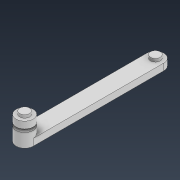
# Autodesk Inventor part: Support
Saved by Autodesk Inventor 2021 (Build 250183000, 183)
## iProperties
Created: 2021-01-30
Part Number: Support
Material: Generic
Document SubType Name: Modeling
Designer: PaisW
Density: 1 g/cm^3
Appearance: Default
Author: PaisW
Autodesk Inventor part; units mm, degrees
ref_plane "YZ Plane" through (0, 0, 0) normal (1, 0, 0) x (0, 1, 0)
ref_plane "XZ Plane" through (0, 0, 0) normal (0, 1, 0) x (-1, 0, 0)
ref_plane "XY Plane" through (0, 0, 0) normal (0, 0, 1) x (1, 0, 0)
sketch "Sketch1" plane through (0, 0, 0) normal (0, 1, 0) x (-1, 0, 0)
  line L0 (26.15, 200) -> (-26.15, 200)
  line L1 (-26.15, 200) -> (-26.15, -200)
  line L2 (-26.15, -200) -> (26.15, -200)
  line L3 (26.15, -200) -> (26.15, 200)
  circle A0 centre (0, 200) radius 26.15
  circle A1 centre (0, -200) radius 26.15
  point P0 (0, 0)
  point P1 (26.15, 0)
  point P2 (26.15, 200)
  point P3 (26.15, -200)
  dimension "d0" = 52.3
  dimension "d1" = 400
  constraints: 8 end point, 3 midpoint, 2 parallel, 1 coincident, 1 horizontal, 1 horizontal alignment, 1 perpendicular, 1 vertical alignment, 6 other
  measures "d0" distance between parallel lines of L1 L3
  measures "d1" distance between parallel lines of L0 L2
extrude "Extrusion1" add sketch "Sketch1" along normal blind 38.8
sketch "Sketch2" plane through (0, 38.8, 0) normal (0, 1, 0) x (1, 0, 0)
  line L0 (26.15, -200) -> (26.15, 200) projected
  circle A0 centre (0, -200) radius 26.15
  arc A1 (-26.15, -200) -> (26.15, -200) centre (0, -200) ccw projected
  circle A2 centre (0, 200) radius 26.15
  arc A3 (26.15, 200) -> (-26.15, 200) centre (0, 200) ccw projected
  line L1 (-26.15, -200) -> (-26.15, 200)
  line L2 (26.15, 200) -> (26.15, -200)
  circle A4 centre (0, 200) radius 15
  point P0 (0, 0)
  dimension "d6" = 30
  constraints: 4 end point, 3 centre point, 2 concentric, 2 point on circle, 1 coincident, 1 horizontal alignment, 1 parallel, 1 tangent, 1 vertical
  measures "d6" diameter of A4
extrude "Extrusion2" cut sketch "Sketch2" against normal blind 9.3
sketch "Sketch3" plane through (0, 0, 0) normal (0, -1, 0) x (1, 0, 0)
  circle A0 centre (0, -200) radius 26.15
  arc A1 (-26.15, -200) -> (26.15, -200) centre (0, -200) ccw projected
  arc A2 (26.15, 200) -> (-26.15, 200) centre (0, 200) ccw projected
  circle A3 centre (0, 350) radius 26.15
  circle A4 centre (0, -200) radius 15
  line L0 (-26.15, -200) -> (-26.15, 200) projected
  line L1 (-26.15, -200) -> (-26.15, 200)
  arc A5 (26.15, 200) -> (-26.15, 200) centre (0, 200) ccw projected
  line L2 (26.15, 200) -> (26.15, -200)
  point P0 (0, 0)
  point P1 (-26.15, -200)
  point P2 (26.15, -200)
  dimension "d10" = 30
  constraints: 4 end point, 3 vertical, 2 centre point, 2 coincident, 2 concentric, 1 horizontal alignment, 1 tangent, 3 other
  measures "d10" diameter of A4
extrude "Extrusion3" cut sketch "Sketch3" against normal blind 9 contours A0 | A0 L0 A2 L2
sketch "Sketch7" plane through (0, 29.5, 0) normal (0, 1, 0) x (1, 0, 0)
  circle A0 centre (0, -200) radius 26.15
  arc A1 (-26.15, -200) -> (26.15, -200) centre (0, -200) ccw projected
  point P0 (0, 0)
  constraints: 2 concentric, 1 centre point
extrude "Extrusion6" add sketch "Sketch7" along normal blind 21.1
sketch "Sketch8" plane through (0, 50.6, 200) normal (0, 1, 0) x (1, 0, 0)
  circle A0 centre (0, 0) radius 15
  circle A1 centre (0, 0) radius 26.15 projected
  point P0 (0, 200)
  dimension "d21" = 30
  constraints: 1 centre point, 1 concentric
  measures "d21" diameter of A0
extrude "Extrusion7" add sketch "Sketch8" along normal blind 9.3 contours A0
sketch "Sketch9" plane through (0, 59.9, 200) normal (0, 1, 0) x (1, 0, 0)
  circle A0 centre (0, 0) radius 26.15
  circle A1 centre (0, 0) radius 15 projected
  circle A2 centre (0, 0) radius 26.15 projected
  point P0 (0, 200)
  constraints: 2 concentric, 1 centre point
extrude "Extrusion8" add sketch "Sketch9" along normal blind 20.8 contours A0 | A1
sketch "Sketch10" plane through (0, 80.7, 200) normal (0, 1, 0) x (1, 0, 0)
  circle A0 centre (0, 0) radius 15
  circle A1 centre (0, 0) radius 15 projected
  circle A2 centre (0, 0) radius 26.15 projected
  point P0 (0, 200)
  constraints: 2 concentric, 1 centre point
extrude "Extrusion9" add sketch "Sketch10" along normal blind 9 contours A0
body "Solid1"
